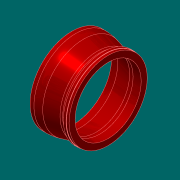
# Autodesk Inventor part: A1-19027-400-10 HCWI liner - reducer
Saved by Autodesk Inventor 2017.3 (Build 213257000, 257)
## iProperties
Created: 2019-08-16
Part Number: A1-19027-400-10 HCWI liner - reducer
Material: Iron, HCWI
Document SubType Name: Modeling
Designer: GVD
Density: 7.33517 g/cm^3
Appearance: Iron Gray(1)
Mass: 503749 g
Surface Area: 40346.3 cm^2
Volume: 68675.8 cm^3
Description: 28 1/2" ID x 24 1/2" ID x 1 1/2" WALL x 13 15/32" HCWI REDUCER, ASTM A532 CLASS III TYPE A, PF#(TBD)
Author: GVD
Autodesk Inventor part; units mm, degrees
ref_plane "YZ Plane" through (0, 0, 0) normal (1, 0, 0) x (0, 1, 0)
ref_plane "XZ Plane" through (0, 0, 0) normal (0, 1, 0) x (-1, 0, 0)
ref_plane "XY Plane" through (0, 0, 0) normal (0, 0, 1) x (1, 0, 0)
sketch "Sketch1" plane through (0, 0, 0) normal (0, 0, 1) x (1, 0, 0)
  line L0 (0, 0) -> (341.7, 0)
  line L1 (0, 361.95) -> (6.0161, 361.95)
  arc A0 (79.941, 352.8494) -> (6.0161, 361.95) centre (6.0161, 57.15) ccw
  line L2 (79.941, 352.8494) -> (228.5376, 315.7003)
  arc A1 (228.5376, 315.7003) -> (265.5, 311.15) centre (265.5, 463.55) ccw
  line L3 (265.5, 311.15) -> (341.7, 311.15)
  line L4 (341.7, 311.15) -> (341.7, 342.9)
  line L5 (341.7, 342.9) -> (314.3516, 342.9)
  arc A2 (240.4268, 352.0006) -> (314.3516, 342.9) centre (314.3516, 647.7) ccw
  line L6 (240.4268, 352.0006) -> (110.0313, 384.5994)
  arc A3 (110.0313, 384.5994) -> (36.1064, 393.7) centre (36.1064, 88.9) ccw
  line L7 (36.1064, 393.7) -> (0, 393.7)
  line L8 (0, 393.7) -> (0, 361.95)
  dimension "d0" = 341.7
  dimension "d1" = 723.9
  dimension "d2" = 31.75
  dimension "d3" = 622.3
  dimension "d4" = 304.8
  dimension "d5" = 152.4
  dimension "d6" = 304.8
  dimension "d7" = 304.8
  dimension "d8" = 38.1
  dimension "d9" = 31.75
  dimension "d10" = 76.2
  dimension "d12" = 14.036
  constraints: 18 end point, 8 point on circle, 8 tangent, 4 centre point, 3 horizontal, 3 perpendicular, 2 parallel, 2 point on line
  measures "d0" distance of L0.start L0.end
  measures "d1" diameter of L1 L0
  measures "d2" distance of L7.end L1.start
  measures "d3" diameter of L3 L0
  measures "d4" radius of A0
  measures "d5" radius of A1
  measures "d6" radius of A3
  measures "d7" radius of A2
  measures "d8" distance between parallel lines of L2 L6
  measures "d9" distance of L3.end L4.end
  measures "d10" distance of L3.start L3.end
  measures "d12" angle of L2 L1
revolve "Revolution1" add sketch "Sketch1" angle 360 about axis through (0, 0, 0) along (1, 0, 0)
sketch "Sketch2" plane through (0, 0, 0) normal (-1, 0, 0) x (0, 0, 1)
  circle A0 centre (0, 0) radius 381
  dimension "d14" = 762
  constraints: 1 centre point, 1 coincident
  measures "d14" diameter of A0
extrude "Extrusion1" cut sketch "Sketch2" against normal blind 12.7
sketch "Sketch3" plane through (341.7, 0, 0) normal (1, 0, 0) x (0, 0, -1)
  circle A0 centre (0, 0) radius 342.9 projected
  circle A1 centre (0, 0) radius 371.475
  dimension "d17" = 742.95
  constraints: 1 centre point, 1 coincident
  measures "d17" diameter of A1
extrude "Extrusion2" add sketch "Sketch3" against normal blind 50.8
sketch "Sketch4" plane through (341.7, 0, 0) normal (1, 0, 0) x (0, 0, -1)
  circle A0 centre (0, 0) radius 371.475 projected
  circle A1 centre (0, 0) radius 368.046
  dimension "d27" = 736.092
  constraints: 1 centre point, 1 coincident
  measures "d27" diameter of A1
extrude "Extrusion3" cut sketch "Sketch4" against normal blind 25.4
fillet "Fillet1" radius 0.7937 2 edges at (12.7, 0, -381) (316.3, 0, 368.046)
chamfer "Chamfer1" distance 0.7937 angle 45 1 edges at (0, 0, -381)
fillet "Fillet2" radius 25.4 1 edges at (290.9, -343.8035, 0)
equation "\"d9\" = d2"
body "Solid1"
